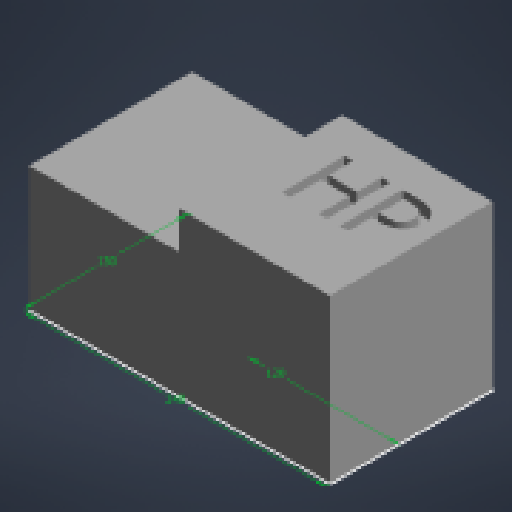
# Autodesk Inventor part: HotPlate
Saved by Autodesk Inventor 2024.2 (Build 282272000, 272)
## iProperties
Created: 2024-10-04
Part Number: HotPlate
Material: Generic
Document SubType Name: Modeling
Designer: jerem
Density: 1 g/cm^3
Appearance: Default
Author: jerem
Autodesk Inventor part; units mm, degrees
ref_plane "YZ Plane" through (0, 0, 0) normal (1, 0, 0) x (0, 1, 0)
ref_plane "XZ Plane" through (0, 0, 0) normal (0, 1, 0) x (-1, 0, 0)
ref_plane "XY Plane" through (0, 0, 0) normal (0, 0, 1) x (1, 0, 0)
sketch "Sketch1" plane through (0, 0, 0) normal (0, 1, 0) x (-1, 0, 0)
  line L0 (-120, -65) -> (120, -65)
  line L1 (120, -65) -> (120, 65)
  line L2 (120, 65) -> (-120, 65)
  line L3 (-120, 65) -> (-120, -65)
  line L4 (-120, -65) -> (120, 65) construction
  line L5 (120, -65) -> (-120, 65) construction
  line L6 (0, 65) -> (0, -65)
  point P0 (0, 0)
  dimension "d0" = 240
  dimension "d1" = 130
  dimension "d4" = 120
  constraints: 14 end point, 4 midpoint, 2 parallel, 2 perpendicular, 1 horizontal
  measures "d0" distance of L2.end L1.end
  measures "d1" distance of L1.end L0.end
  measures "d4" distance between parallel lines of L6 L3
extrude "Extrusion1" add sketch "Sketch1" along normal blind 100
extrude "Extrusion2" add sketch "Sketch1" along normal blind 30 from surface at 100 contours L3 L2 L6 L0
sketch "Sketch2" plane through (0, 130, -65) normal (0, 1, 0) x (1, 0, 0)
  line L0 (24.228, -27.798) -> (40.6948, -27.798) construction
  line L1 (40.6948, -27.798) -> (40.6948, -38.1545) construction
  line L2 (40.6948, -38.1545) -> (24.228, -38.1545) construction
  line L3 (24.228, -38.1545) -> (24.228, -27.798) construction
  line L4 (65.5975, -77.798) -> (58.9525, -77.798)
  line L5 (58.9525, -77.798) -> (58.9525, -53.3247)
  line L6 (58.9525, -53.3247) -> (35.9379, -53.3247)
  line L7 (35.9379, -53.3247) -> (35.9379, -77.798)
  line L8 (35.9379, -77.798) -> (29.2928, -77.798)
  line L9 (29.2928, -77.798) -> (29.2928, -27.798)
  line L10 (29.2928, -27.798) -> (35.9379, -27.798)
  line L11 (35.9379, -27.798) -> (35.9379, -47.409)
  line L12 (35.9379, -47.409) -> (58.9525, -47.409)
  line L13 (58.9525, -47.409) -> (58.9525, -27.798)
  line L14 (58.9525, -27.798) -> (65.5975, -27.798)
  line L15 (65.5975, -27.798) -> (65.5975, -77.798)
  spline S0 degree 2 poles (107.3317, -42.8709) (107.3317, -46.1124) (105.0222, -51.9471) (102.9557, -53.973) knots 0 0 0 1 2 2 2
  spline S1 degree 2 poles (102.9557, -53.973) (100.3625, -56.5257) (93.3528, -59.1594) (88.0043, -59.1594) knots 0 0 0 1 2 2 2
  line L16 (88.0043, -59.1594) -> (82.3723, -59.1594)
  line L17 (82.3723, -59.1594) -> (82.3723, -77.798)
  line L18 (82.3723, -77.798) -> (75.7272, -77.798)
  line L19 (75.7272, -77.798) -> (75.7272, -27.798)
  line L20 (75.7272, -27.798) -> (88.288, -27.798)
  spline S2 degree 2 poles (88.288, -27.798) (92.745, -27.798) (98.9849, -29.2566) (101.3755, -30.9179) knots 0 0 0 1 2 2 2
  spline S3 degree 2 poles (101.3755, -30.9179) (104.1713, -32.8223) (107.3317, -38.6975) (107.3317, -42.8709) knots 0 0 0 1 2 2 2
  spline S4 degree 2 poles (100.403, -43.0735) (100.403, -40.4803) (98.6202, -36.6715) (96.7969, -35.456) knots 0 0 0 1 2 2 2
  spline S5 degree 2 poles (96.7969, -35.456) (95.2167, -34.4025) (91.0027, -33.5516) (87.8828, -33.5516) knots 0 0 0 1 2 2 2
  line L21 (87.8828, -33.5516) -> (82.3723, -33.5516)
  line L22 (82.3723, -33.5516) -> (82.3723, -53.4868)
  line L23 (82.3723, -53.4868) -> (86.9103, -53.4868)
  spline S6 degree 2 poles (86.9103, -53.4868) (90.9622, -53.4868) (95.946, -52.1902) (97.5667, -50.4884) knots 0 0 0 1 2 2 2
  spline S7 degree 2 poles (97.5667, -50.4884) (99.0659, -48.9892) (100.403, -45.4641) (100.403, -43.0735) knots 0 0 0 1 2 2 2
  point P0 (0, -65)
  point P1 (67.1766, -110.0367)
  constraints: 2 other
extrude "Extrusion3" cut sketch "Sketch2" against normal blind 10
body "Solid1"
